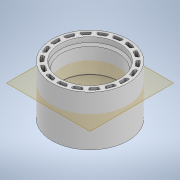
# Autodesk Inventor part: Kolo_v3
Saved by Autodesk Inventor 2020 (Build 240168000, 168)
## iProperties
Created: 2019-12-28
Part Number: Kolo_v3
Material: Generic
Document SubType Name: Modeling
Designer: atmat
Density: 1 g/cm^3
Appearance: Default
Author: atmat
Autodesk Inventor part; units mm, degrees
ref_plane "YZ Plane" through (0, 0, 0) normal (1, 0, 0) x (0, 1, 0)
ref_plane "XZ Plane" through (0, 0, 0) normal (0, 1, 0) x (-1, 0, 0)
ref_plane "XY Plane" through (0, 0, 0) normal (0, 0, 1) x (1, 0, 0)
sketch "Sketch1" plane through (0, 0, 0) normal (0, 1, 0) x (-1, 0, 0)
  circle A0 centre (0, 0) radius 19
  circle A1 centre (0, 0) radius 15
  dimension "d0" = 38
  dimension "d1" = 30
  constraints: 2 centre point, 2 coincident
  measures "d0" diameter of A0
  measures "d1" diameter of A1
extrude "Extrusion1" add sketch "Sketch1" along normal blind 25
ref_plane "Work Plane1" through (0, 15.5, 0) normal (0, 1, 0) x (1, 0, 0)
sketch "Sketch2" plane through (0, 15.5, 0) normal (0, 1, 0) x (1, 0, 0)
  circle A0 centre (0, 0) radius 15
  circle A1 centre (0, 0) radius 14
  dimension "d5" = 28
  constraints: 2 centre point, 2 coincident
  measures "d5" diameter of A1
extrude "Extrusion2" add sketch "Sketch2" along normal blind 7 and the other way blind 7
chamfer "Chamfer1" distance 1 angle 45 2 edges at (-14, 22.5, 0) (-14, 8.5, 0)
sketch "Sketch3" plane through (0, 0, 0) normal (0, -1, 0) x (1, 0, 0)
  arc A0 (17.6412, -2.3723) -> (17.6412, 2.3723) centre (0, 0) ccw
  arc A1 (16.1304, -1.5) -> (16.1304, 1.5) centre (0, 0) ccw
  circle A2 centre (0, 0) radius 15 projected
  line L0 (17.6412, -2.3723) -> (16.1304, -1.5)
  line L1 (16.1304, 1.5) -> (17.6412, 2.3723)
  line L2 (18.7691, 0) -> (11.9542, 0) construction
  circle A3 centre (0, 0) radius 19 projected
  dimension "d15" = 30
  dimension "d16" = 30
  dimension "d17" = 1.2
  dimension "d18" = 1.2
  dimension "d19" = 3
  dimension "d20" = 1.5
  dimension "d21" = 0
  constraints: 6 end point, 4 point on circle, 2 centre point, 2 concentric, 1 horizontal
  measures "d15" angle of L2 L0
  measures "d16" angle of L1 L2
  measures "d17" radial gap between concentric circles of A3 A0
  measures "d18" radial gap between concentric circles of A2 A1
  measures "d19" distance of L1.start L0.end
  measures "d20" distance from line of L2 L0.end
  measures "d21" distance from line of point (0, 0) L2
extrude "Extrusion3" cut sketch "Sketch3" against normal blind 25 contours L0 A1 L1 A0
fillet "Fillet1" radius 0.4 4 edges at (17.6412, 12.5, -2.3723) (16.1304, 12.5, -1.5) (16.1304, 12.5, 1.5) (17.6412, 12.5, 2.3723)
pattern_circular "Circular Pattern1" count 18 over 360 about axis through (0, -10, 0) along (0, 1, 0) of "Fillet1", "Extrusion3"
body "Solid1"
